Autodesk Inventor part; units mm, degrees
(part 3 of 3)
  line L498 (-0.5393, -47.9465) -> (-0.5393, -47.9687)
  line L499 (-0.5393, -47.9687) -> (-0.9592, -47.9687)
  spline S529 degree 2 poles (-0.9592, -47.9687) (-0.9864, -47.902) (-1.0654, -47.6995) (-1.0876, -47.6204) knots 0 0 0 1 2 2 2
  spline S530 degree 2 poles (-1.0876, -47.6204) (-1.1198, -47.5093) (-1.1519, -47.3265) (-1.1519, -47.1882) knots 0 0 0 1 2 2 2
  spline S531 degree 2 poles (0.298, -47.6353) (0.4536, -47.6303) (0.6809, -47.5661) (0.7575, -47.5044) knots 0 0 0 1 2 2 2
  spline S532 degree 2 poles (0.7575, -47.5044) (0.8439, -47.4377) (0.9353, -47.2277) (0.9353, -47.0721) knots 0 0 0 1 2 2 2
  spline S533 degree 2 poles (0.9353, -47.0721) (0.9353, -46.919) (0.8439, -46.7041) (0.755, -46.6151) knots 0 0 0 1 2 2 2
  spline S534 degree 2 poles (0.755, -46.6151) (0.6636, -46.5287) (0.4438, -46.4398) (0.298, -46.4274) knots 0 0 0 1 2 2 2
  line L500 (0.298, -46.4274) -> (0.298, -47.6353)
  line L501 (0.7747, -49.6137) -> (0.7747, -49.594)
  spline S535 degree 2 poles (0.7747, -49.594) (0.7871, -49.5495) (0.792, -49.4532) (0.792, -49.3865) knots 0 0 0 1 2 2 2
  spline S536 degree 2 poles (0.792, -49.3865) (0.792, -49.2309) (0.6562, -48.9246) (0.5228, -48.7863) knots 0 0 0 1 2 2 2
  line L502 (0.5228, -48.7863) -> (-1.1, -48.7863)
  line L503 (-1.1, -48.7863) -> (-1.1, -48.401)
  line L504 (-1.1, -48.401) -> (1.1872, -48.401)
  line L505 (1.1872, -48.401) -> (1.1872, -48.7863)
  line L506 (1.1872, -48.7863) -> (0.8464, -48.7863)
  spline S537 degree 2 poles (0.8464, -48.7863) (1.0341, -48.9962) (1.1872, -49.3099) (1.1872, -49.4581) knots 0 0 0 1 2 2 2
  spline S538 degree 2 poles (1.1872, -49.4581) (1.1872, -49.5174) (1.1823, -49.5767) (1.1749, -49.6137) knots 0 0 0 1 2 2 2
  line L507 (1.1749, -49.6137) -> (0.7747, -49.6137)
  spline S539 degree 2 poles (-1.4656, -49.9941) (-1.4829, -50.0336) (-1.5372, -50.1843) (-1.5594, -50.2806) knots 0 0 0 1 2 2 2
  spline S540 degree 2 poles (-1.5594, -50.2806) (-1.5866, -50.3869) (-1.6187, -50.5672) (-1.6187, -50.6734) knots 0 0 0 1 2 2 2
  spline S541 degree 2 poles (-1.6187, -50.6734) (-1.6187, -50.8512) (-1.5248, -51.0982) (-1.4409, -51.1674) knots 0 0 0 1 2 2 2
  spline S542 degree 2 poles (-1.4409, -51.1674) (-1.3569, -51.2341) (-1.137, -51.2859) (-0.9963, -51.2859) knots 0 0 0 1 2 2 2
  line L508 (-0.9963, -51.2859) -> (-0.7962, -51.2859)
  spline S543 degree 2 poles (-0.7962, -51.2859) (-0.932, -51.1303) (-1.0605, -50.8315) (-1.0605, -50.6067) knots 0 0 0 1 2 2 2
  spline S544 degree 2 poles (-1.0605, -50.6067) (-1.0605, -50.2164) (-0.48, -49.7545) (0.0658, -49.7545) knots 0 0 0 1 2 2 2
  spline S545 degree 2 poles (0.0658, -49.7545) (0.3499, -49.7545) (0.7896, -49.9151) (0.9452, -50.0485) knots 0 0 0 1 2 2 2
  spline S546 degree 2 poles (0.9452, -50.0485) (1.0909, -50.1769) (1.2515, -50.5301) (1.2515, -50.7178) knots 0 0 0 1 2 2 2
  spline S547 degree 2 poles (1.2515, -50.7178) (1.2515, -50.8957) (1.1675, -51.155) (1.0909, -51.2859) knots 0 0 0 1 2 2 2
  line L509 (1.0909, -51.2859) -> (1.1872, -51.3082)
  line L510 (1.1872, -51.3082) -> (1.1872, -51.6713)
  line L511 (1.1872, -51.6713) -> (-0.8382, -51.6713)
  spline S548 degree 2 poles (-0.8382, -51.6713) (-1.4211, -51.6713) (-1.9645, -51.1649) (-1.9645, -50.6437) knots 0 0 0 1 2 2 2
  spline S549 degree 2 poles (-1.9645, -50.6437) (-1.9645, -50.4758) (-1.9102, -50.125) (-1.8657, -49.9744) knots 0 0 0 1 2 2 2
  line L512 (-1.8657, -49.9744) -> (-1.4656, -49.9744)
  line L513 (-1.4656, -49.9744) -> (-1.4656, -49.9941)
  line L514 (-0.48, -51.2859) -> (0.7772, -51.2859)
  spline S550 degree 2 poles (0.7772, -51.2859) (0.8464, -51.1427) (0.9057, -50.9006) (0.9057, -50.7796) knots 0 0 0 1 2 2 2
  spline S551 degree 2 poles (0.9057, -50.7796) (0.9057, -50.4881) (0.4759, -50.1522) (0.0733, -50.1522) knots 0 0 0 1 2 2 2
  spline S552 degree 2 poles (0.0733, -50.1522) (-0.3071, -50.1522) (-0.7048, -50.4066) (-0.7048, -50.6931) knots 0 0 0 1 2 2 2
  spline S553 degree 2 poles (-0.7048, -50.6931) (-0.7048, -50.8438) (-0.5862, -51.16) (-0.48, -51.2859) knots 0 0 0 1 2 2 2
  spline S554 degree 2 poles (-0.8579, -53.504) (-0.8925, -53.4571) (-1.016, -53.299) (-1.0531, -53.2249) knots 0 0 0 1 2 2 2
  spline S555 degree 2 poles (-1.0531, -53.2249) (-1.1074, -53.1236) (-1.1642, -52.9334) (-1.1642, -52.7605) knots 0 0 0 1 2 2 2
  spline S556 degree 2 poles (-1.1642, -52.7605) (-1.1642, -52.6198) (-1.058, -52.3653) (-0.9617, -52.269) knots 0 0 0 1 2 2 2
  spline S557 degree 2 poles (-0.9617, -52.269) (-0.8678, -52.1776) (-0.5912, -52.0665) (-0.438, -52.0665) knots 0 0 0 1 2 2 2
  spline S558 degree 2 poles (-0.438, -52.0665) (-0.2009, -52.0665) (0.135, -52.2665) (0.2313, -52.4839) knots 0 0 0 1 2 2 2
  spline S559 degree 2 poles (0.2313, -52.4839) (0.3203, -52.6766) (0.387, -53.2002) (0.4042, -53.504) knots 0 0 0 1 2 2 2
  line L515 (0.4042, -53.504) -> (0.4783, -53.504)
  spline S560 degree 2 poles (0.4783, -53.504) (0.6117, -53.504) (0.7772, -53.4225) (0.8241, -53.3484) knots 0 0 0 1 2 2 2
  spline S561 degree 2 poles (0.8241, -53.3484) (0.8711, -53.2743) (0.9007, -53.0619) (0.9007, -52.9483) knots 0 0 0 1 2 2 2
  spline S562 degree 2 poles (0.9007, -52.9483) (0.9007, -52.8149) (0.8217, -52.4543) (0.7451, -52.274) knots 0 0 0 1 2 2 2
  line L516 (0.7451, -52.274) -> (0.7451, -52.2517)
  line L517 (0.7451, -52.2517) -> (1.1378, -52.2517)
  spline S563 degree 2 poles (1.1378, -52.2517) (1.1675, -52.3579) (1.2416, -52.7556) (1.2416, -52.9507) knots 0 0 0 1 2 2 2
  spline S564 degree 2 poles (1.2416, -52.9507) (1.2416, -53.1879) (1.1675, -53.5114) (1.0711, -53.6399) knots 0 0 0 1 2 2 2
  spline S565 degree 2 poles (1.0711, -53.6399) (0.9773, -53.7658) (0.6784, -53.8893) (0.4635, -53.8893) knots 0 0 0 1 2 2 2
  line L518 (0.4635, -53.8893) -> (-1.1, -53.8893)
  line L519 (-1.1, -53.8893) -> (-1.1, -53.504)
  line L520 (-1.1, -53.504) -> (-0.8579, -53.504)
  line L521 (-0.5368, -53.504) -> (0.098, -53.504)
  spline S566 degree 2 poles (0.098, -53.504) (0.0856, -53.3657) (0.0436, -52.9483) (0.0041, -52.8174) knots 0 0 0 1 2 2 2
  spline S567 degree 2 poles (0.0041, -52.8174) (-0.0428, -52.6642) (-0.238, -52.4641) (-0.4109, -52.4641) knots 0 0 0 1 2 2 2
  spline S568 degree 2 poles (-0.4109, -52.4641) (-0.6085, -52.4641) (-0.8085, -52.6864) (-0.8085, -52.8989) knots 0 0 0 1 2 2 2
  spline S569 degree 2 poles (-0.8085, -52.8989) (-0.8085, -53.0792) (-0.6529, -53.3756) (-0.5368, -53.504) knots 0 0 0 1 2 2 2
  spline S570 degree 2 poles (-1.1445, -55.1219) (-1.1445, -54.8082) (-0.7863, -54.455) (-0.3985, -54.455) knots 0 0 0 1 2 2 2
  line L522 (-0.3985, -54.455) -> (0.8686, -54.455)
  line L523 (0.8686, -54.455) -> (0.8686, -54.1956)
  line L524 (0.8686, -54.1956) -> (1.1872, -54.1956)
  line L525 (1.1872, -54.1956) -> (1.1872, -54.455)
  line L526 (1.1872, -54.455) -> (1.8443, -54.455)
  line L527 (1.8443, -54.455) -> (1.8443, -54.8403)
  line L528 (1.8443, -54.8403) -> (1.1872, -54.8403)
  line L529 (1.1872, -54.8403) -> (1.1872, -55.5492)
  line L530 (1.1872, -55.5492) -> (0.8686, -55.5492)
  line L531 (0.8686, -55.5492) -> (0.8686, -54.8403)
  line L532 (0.8686, -54.8403) -> (-0.2207, -54.8403)
  spline S571 degree 2 poles (-0.2207, -54.8403) (-0.3936, -54.8403) (-0.5838, -54.8526) (-0.6653, -54.8946) knots 0 0 0 1 2 2 2
  spline S572 degree 2 poles (-0.6653, -54.8946) (-0.7369, -54.9292) (-0.8085, -55.0848) (-0.8085, -55.2182) knots 0 0 0 1 2 2 2
  spline S573 degree 2 poles (-0.8085, -55.2182) (-0.8085, -55.3121) (-0.7517, -55.4874) (-0.7344, -55.527) knots 0 0 0 1 2 2 2
  line L533 (-0.7344, -55.527) -> (-0.7344, -55.5492)
  line L534 (-0.7344, -55.5492) -> (-1.0802, -55.5492)
  spline S574 degree 2 poles (-1.0802, -55.5492) (-1.1099, -55.4405) (-1.1445, -55.2182) (-1.1445, -55.1219) knots 0 0 0 1 2 2 2
  spline S575 degree 2 poles (-0.8579, -57.1078) (-0.8925, -57.0608) (-1.016, -56.9028) (-1.0531, -56.8287) knots 0 0 0 1 2 2 2
  spline S576 degree 2 poles (-1.0531, -56.8287) (-1.1074, -56.7274) (-1.1642, -56.5372) (-1.1642, -56.3643) knots 0 0 0 1 2 2 2
  spline S577 degree 2 poles (-1.1642, -56.3643) (-1.1642, -56.2235) (-1.058, -55.9691) (-0.9617, -55.8728) knots 0 0 0 1 2 2 2
  spline S578 degree 2 poles (-0.9617, -55.8728) (-0.8678, -55.7814) (-0.5912, -55.6702) (-0.438, -55.6702) knots 0 0 0 1 2 2 2
  spline S579 degree 2 poles (-0.438, -55.6702) (-0.2009, -55.6702) (0.135, -55.8703) (0.2313, -56.0877) knots 0 0 0 1 2 2 2
  spline S580 degree 2 poles (0.2313, -56.0877) (0.3203, -56.2803) (0.387, -56.804) (0.4042, -57.1078) knots 0 0 0 1 2 2 2
  line L535 (0.4042, -57.1078) -> (0.4783, -57.1078)
  spline S581 degree 2 poles (0.4783, -57.1078) (0.6117, -57.1078) (0.7772, -57.0263) (0.8241, -56.9522) knots 0 0 0 1 2 2 2
  spline S582 degree 2 poles (0.8241, -56.9522) (0.8711, -56.8781) (0.9007, -56.6656) (0.9007, -56.552) knots 0 0 0 1 2 2 2
  spline S583 degree 2 poles (0.9007, -56.552) (0.9007, -56.4186) (0.8217, -56.058) (0.7451, -55.8777) knots 0 0 0 1 2 2 2
  line L536 (0.7451, -55.8777) -> (0.7451, -55.8555)
  line L537 (0.7451, -55.8555) -> (1.1378, -55.8555)
  spline S584 degree 2 poles (1.1378, -55.8555) (1.1675, -55.9617) (1.2416, -56.3594) (1.2416, -56.5545) knots 0 0 0 1 2 2 2
  spline S585 degree 2 poles (1.2416, -56.5545) (1.2416, -56.7916) (1.1675, -57.1152) (1.0711, -57.2436) knots 0 0 0 1 2 2 2
  spline S586 degree 2 poles (1.0711, -57.2436) (0.9773, -57.3696) (0.6784, -57.4931) (0.4635, -57.4931) knots 0 0 0 1 2 2 2
  line L538 (0.4635, -57.4931) -> (-1.1, -57.4931)
  line L539 (-1.1, -57.4931) -> (-1.1, -57.1078)
  line L540 (-1.1, -57.1078) -> (-0.8579, -57.1078)
  line L541 (-0.5368, -57.1078) -> (0.098, -57.1078)
  spline S587 degree 2 poles (0.098, -57.1078) (0.0856, -56.9695) (0.0436, -56.552) (0.0041, -56.4211) knots 0 0 0 1 2 2 2
  spline S588 degree 2 poles (0.0041, -56.4211) (-0.0428, -56.268) (-0.238, -56.0679) (-0.4109, -56.0679) knots 0 0 0 1 2 2 2
  spline S589 degree 2 poles (-0.4109, -56.0679) (-0.6085, -56.0679) (-0.8085, -56.2902) (-0.8085, -56.5026) knots 0 0 0 1 2 2 2
  spline S590 degree 2 poles (-0.8085, -56.5026) (-0.8085, -56.6829) (-0.6529, -56.9793) (-0.5368, -57.1078) knots 0 0 0 1 2 2 2
  point P0 (-58, 0)
  point P1 (58, 0)
  point P2 (-0.2479, 27.0589)
  point P3 (-0.2479, -57.7549)
  point P4 (-0.2479, 57.7549)
  dimension "d53" = 12
  dimension "d54" = 12
  dimension "d56" = 12.5
  dimension "d57" = 12.5
  dimension "d55" = 25
  constraints: 5 coincident, 5 midpoint, 3 collinear, 2 horizontal alignment, 2 point on line, 1 centre point, 1 parallel, 18 other
  measures "d55" diameter of A4
extrude "Estrusione2" cut sketch "Schizzo5" against normal blind 1 contours L255 L256 L249 L13 | L13 L249 L250 L251 L252 L253 L254 L255 | S230 S231 L13 S236 S237 | L13 S237 S234 S235 S236 S231 S232 S233 S230 | L258 L259 L260 L13 | L13 L260 L261 L262 S240 S241 L263 L257 S238 S239 L258 | L264 L265 L266 L13 L268 L269 | L13 L269 L270 L264 | S246 S247 S248 L273 L274 S249 S250 S242 L13 | L13 S242 S243 S244 S245 L271 L272 S246 | L277 L278 L279 L13 | L13 L279 L280 L281 S257 S258 L282 L276 S255 S256 L277 | L286 S268 S269 L287 L288 S259 S260 S261 S262 L283 S263 S264 L13 S272 S273 L289 | L13 L289 S270 S271 S272 S264 S265 S266 S267 L284 L285 L286 | L293 L294 L295 S274 S275 S276 S277 S278 L13 S287 S288 S289 L296 | L13 L296 S286 S287 S278 S279 L290 S280 S281 S282 L291 L292 S283 S284 S285 L293 | L307 S291 S292 S293 L308 L309 S294 S290 L297 L13 | L13 L297 L298 L299 L300 L301 L302 L303 L304 L305 L306 L307 | L313 L314 L315 S295 S296 S297 S298 S299 L13 S308 S309 S310 L316 | L13 L316 S307 S308 S299 S300 L310 S301 S302 S303 L311 L312 S304 S305 S306 L313 | S579 S580 L535 S581 S582 S583 L536 L537 S584 S585 S586 L538 L13 L541 S587 S588 | L13 S588 S589 S590 L541 L538 L539 L540 S575 S576 S577 S578 S579 | L522 L523 L524 L525 L526 L527 L528 L529 L530 L531 L532 L13 | L13 L532 S571 S572 S573 L533 L534 S574 S570 L522 | S558 S559 L515 S560 S561 S562 L516 L517 S563 S564 S565 L518 L13 L521 S566 S567 | L13 S567 S568 S569 L521 L518 L519 L520 S554 S555 S556 S557 S558 | S544 S545 S546 S547 L509 L510 L511 L13 L514 S550 S551 S552 | L13 S552 S553 L514 L511 S548 S549 L512 L513 S539 S540 S541 S542 L508 S543 S544 | L504 L505 L506 S537 S538 L507 L501 S535 S536 L502 L13 | L13 L502 L503 L504 | S522 S523 S524 S525 L496 L497 S526 L13 | L13 S526 S527 S528 L498 L499 S529 S530 S522 | L491 L492 L493 L13 | L13 L493 L494 L489 L490 L491 | L485 L486 L487 S520 S521 L488 L482 S518 S519 L483 L13 | L13 L483 L484 L485 | S511 S512 S513 S510 L13 S517 S514 S515 S516 | L13 S516 S517 S510 S511 | L474 L475 L476 L477 L478 L479 L480 L13 | L13 L480 L481 L474 | L494 L495 L489 L13 | L13 L266 L267 L268 | L18 L19 L20 L21 L22 L23 L24 L25 | L29 L30 L31 L32 | L33 S0 S1 L34 L35 L36 L37 L38 L39 L40 L41 L42 L43 L44 S2 S3 L45 | S4 S5 S6 S7 S8 S9 L46 S10 S11 S12 L47 L48 S13 S14 S15 L49 L50 L51 | L53 L54 S20 S21 S22 L55 L56 L57 L58 L59 S23 S24 L60 | S25 S26 S27 S28 | L61 L62 L63 L64 L65 L66 L67 L68 L69 L70 L71 L72 | L73 S33 S34 S35 S36 L74 L75 L76 S37 S38 S39 L77 L78 L79 L80 L81 S40 S41 S42 S43 S44 L82 L83 | S45 S46 S47 S48 S49 S50 L84 S51 S52 S53 L85 L86 S54 S55 S56 L87 L88 L89 | L91 L92 S61 S62 S63 L93 L94 L95 L96 L97 S64 S65 L98 | L99 L100 S66 S67 S68 L101 L102 L103 S69 S70 S71 L104 L105 L106 | S72 S73 S74 S75 L107 L108 S76 S77 S78 L109 L110 S79 S80 | L112 L113 L114 L115 | S85 S86 S87 S88 L116 L117 S89 S90 S91 L118 L119 S92 S93 | S98 S99 L121 L122 L123 S100 S101 S102 L124 S103 | S112 S113 S114 S115 S116 S117 L131 S118 S119 S120 L132 L133 S121 S122 S123 L134 L135 L136 | L138 L139 S128 S129 S130 S131 S132 S133 S134 L140 L141 L142 | S139 S140 S141 S142 S143 S144 L144 S145 S146 S147 L145 L146 S148 S149 S150 L147 L148 L149 | L151 L152 L153 L154 | S155 S156 S157 S158 S159 S160 L155 S161 S162 S163 L156 L157 S164 S165 S166 L158 L159 L160 | L162 S171 S172 S173 S174 L163 L164 L165 S175 S176 S177 L166 L167 L168 L169 L170 S178 S179 S180 S181 S182 L171 L172 | S183 S184 S185 S186 L173 L174 S187 S188 S189 L175 L176 S190 S191 | L178 L179 S196 S197 S198 L180 L181 L182 L183 L184 S199 S200 L185 | S201 L186 L187 L188 L189 L190 L191 L192 L193 L194 L195 L196 S202 S203 S204 L197 L198 S205 | L199 L200 L201 L202 | L203 L204 L205 L206 | L207 L208 L209 L210 L211 L212 L213 L214 L215 L216 | L217 L218 L219 L220 | L221 L222 L223 L224 | L225 L226 L227 L228 | L229 L230 L231 L232 | L233 L234 L235 L236 | S206 S207 L237 L238 L239 L240 L241 S208 S209 | S214 S215 L243 L244 L245 L246 L247 S216 S217 | S222 S223 S224 S225 | S311 L317 L318 S312 S313 S314 S315 S316 S317 S318 S319 L319 L320 S320 S321 S322 S323 S324 S325 S326 | S327 S328 S329 S330 | S335 S336 S337 S338 S339 L321 L322 S340 S341 S342 S343 S344 L323 L324 S345 S346 | S347 S348 S349 S350 S351 L325 L326 S352 S353 S354 S355 S356 L327 L328 S357 S358 | L329 L330 L331 L332 | L333 L334 L335 L336 | S359 S360 S361 S362 | L337 L338 L339 L340 L341 L342 | S367 S368 S369 S370 L343 L344 S371 S372 S373 L345 L346 S374 S375 | S380 S381 S382 S383 | L348 L349 S388 S389 S390 L350 L351 L352 L353 L354 S391 S392 L355 | S393 S394 S395 S396 S397 S398 L356 S399 S400 S401 L357 L358 S402 S403 S404 L359 L360 L361 | L363 S409 S410 L364 L365 L366 L367 L368 S411 S412 L369 | L370 L371 S413 S414 S415 S416 S417 S418 S419 L372 L373 L374 | S424 S425 S426 S427 | L376 L377 L378 L379 L380 L381 L382 | L383 L384 L385 L386 | L387 L388 L389 L390 | S432 L391 L392 L393 L394 L395 L396 L397 L398 L399 L400 L401 S433 S434 S435 L402 L403 S436 | S437 L404 L405 L406 L407 L408 L409 L410 L411 L412 L413 L414 S438 S439 S440 L415 L416 S441 | L417 L418 L419 L420 | L421 L422 L423 L424 | S442 S443 S444 S445 S446 S447 L425 L426 S448 S449 S450 S451 S452 S453 L427 L428 L429 L430 L431 S454 S455 | S456 S457 S458 S459 S460 S461 L432 S462 S463 S464 L433 L434 S465 S466 S467 L435 L436 L437 | S472 S473 L439 L440 L441 L442 L443 S474 S475 | L445 S480 S481 L446 L447 L448 L449 L450 S482 S483 L451 | L452 L453 L454 L455 | L456 L457 L458 L459 | S484 S485 S486 S487 L460 L461 S488 S489 S490 L462 L463 S491 S492 | L465 L466 L467 L468 | S497 S498 S499 S500 L469 L470 S501 S502 S503 L471 L472 S504 S505
